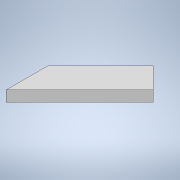
# Autodesk Inventor part: Helenowiak_podpora
Saved by Autodesk Inventor 2021 (Build 250183000, 183)
## iProperties
Created: 2021-03-30
Part Number: Helenowiak_podpora
Material: Ogólny
Document SubType Name: Modeling
Designer: jakub
Density: 1 g/cm^3
Appearance: Domyślna
Author: jakub
Autodesk Inventor part; units mm, degrees
ref_plane "YZ Plane" through (0, 0, 0) normal (1, 0, 0) x (0, 1, 0)
ref_plane "XZ Plane" through (0, 0, 0) normal (0, 1, 0) x (-1, 0, 0)
ref_plane "XY Plane" through (0, 0, 0) normal (0, 0, 1) x (1, 0, 0)
sketch "Szkic3" plane through (0, 0, 0) normal (0, 1, 0) x (-1, 0, 0)
  line L0 (0, 0) -> (-20, 0)
  line L1 (-20, 0) -> (-20, -20)
  line L2 (-20, -20) -> (0, -20)
  line L3 (0, -20) -> (0, 0)
  dimension "d6" = 20
  dimension "d7" = 20
  constraints: 8 end point, 2 parallel, 1 horizontal, 1 perpendicular
  measures "d6" distance of L2.end L1.end
  measures "d7" distance of L1.end L0.end
extrude "Wyciągnięcie proste3" add sketch "Szkic3" along normal blind 5
sketch "Szkic4" plane through (0, 0, 0) normal (0, -1, 0) x (1, 0, 0)
  line L0 (0, 0) -> (20, 0) projected
  line L1 (20, 0) -> (20, -20) projected
  line L2 (0, 0) -> (20, -20)
  line L3 (20, -20) -> (20, 0)
  line L4 (20, 0) -> (0, 0)
  constraints: 6 end point, 1 collinear, 1 perpendicular
extrude "Wyciągnięcie proste4" cut sketch "Szkic4" against normal blind 5
sketch "Szkic5" plane through (0, 5, 0) normal (0, 1, 0) x (1, 0, 0)
  line L0 (20, 20) -> (0, 20) projected
  line L1 (0, 20) -> (25.3553, 45.3553)
  line L2 (0, 20) -> (35.8579, 20) construction
  line L3 (0, 0) -> (20, 20) projected
  line L4 (0, 0) -> (35.3553, 35.3553)
  line L5 (0, 0) -> (50, 0) construction
  line L6 (10.8927, 30.8927) -> (33.735, 53.735)
  line L7 (10.8927, 30.8927) -> (43.1966, 30.8927) construction
  line L8 (35.3553, 35.3553) -> (25.3553, 45.3553)
  dimension "d12" = 45
  dimension "d13" = 50
  dimension "d14" = 45
  dimension "d15" = 45
  constraints: 14 end point, 3 equal length, 3 horizontal, 1 collinear, 1 perpendicular, 1 point on line
  measures "d12" angle of L2 L1
  measures "d13" distance of L3.start L4.end
  measures "d14" angle of L5 L4
  measures "d15" angle of L7 L6
extrude "Wyciągnięcie proste5" add sketch "Szkic5" against normal blind 5
